Autodesk Fusion 360 part; units mm, degrees
(part 2 of 2)
extrude "Extrusion16" cut sketch "Esquisse2" along normal blind 100 contours L1 L2 L3 L4 A0 A1 A2 A3 | L9 L10 L11 L12 bodies 1 2
extrude "Extrusion17" add sketch "Esquisse3" against normal blind 1.4 contours L0 L1 L2 L3 | A0 L4 A1 L5 A2 L6 A3 L7 L288 L289 L290 L291 | A2 A6 | L8 L9 L10 L11 | L12 L13 L14 L15 | L16 L17 L18 L19 | L20 L21 L22 L23 | L24 L25 L26 L27 | L28 L29 L30 L31 | L32 L33 L34 L35 | L36 L37 L38 L39 | L40 L41 L42 L43 | L44 L45 L46 L47 | L48 L49 L50 L51 | L52 L53 L54 L55 | L56 L57 L58 L59 | L60 L61 L62 L63 | L64 L65 L66 L67 | L68 L69 L70 L71 | L72 L73 L74 L75 | L76 L77 L78 L79 | L80 L81 L82 L83 | L84 L85 L86 L87 | L88 L89 L90 L91 | L92 L93 L94 L95 | L96 L97 L98 L99 | L100 L101 L102 L103 | L104 L105 L106 L107 | L108 L109 L110 L111 | L112 L113 L114 L115 | L116 L117 L118 L119 | L120 L121 L122 L123 | L124 L125 L126 L127 | L128 L129 L130 L131 | L132 L133 L134 L135 | L136 L137 L138 L139 | L140 L141 L142 L143 | L144 L145 L146 L147 | L148 L149 L150 L151 | L152 L153 L154 L155 | L156 L157 L158 L159 | L160 L161 L162 L163 | L164 L165 L166 L167 | L168 L169 L170 L171 | L172 L173 L174 L175 | L176 L177 L178 L179 | L180 L182 L183 A9 | L180 A9 | L180 L182 A9 | L180 L181 L182 A9 | L182 A9 | L184 L185 L186 L187 | L188 L189 L190 L191 | L192 L193 L194 L195 | L196 L197 L198 L199 | L200 L201 L202 L203 | L204 L205 L206 L207 L208 L209 L210 L211 | L212 L213 L214 L215 | L216 L218 L219 A8 | L216 A8 | L216 L218 A8 | L216 L217 L218 A8 | L218 A8 | L220 L221 L222 L223 | L224 L225 L226 L227 | L228 L229 L230 L231 | L232 L233 L234 L235 | L236 L237 L238 L239 | L240 L241 L242 L243 | L244 L245 L246 L247 | L248 L249 L250 L251 | L252 L253 L254 L255 | L256 L257 L258 L259 | L260 L261 L262 L263 | L264 L265 L266 L267 | L268 L269 L270 L271 | L272 L273 L274 L275 | L276 L277 L278 L279 | L280 L281 L282 L283 | L284 L285 L286 L287 | A10 | A11 bodies 2
sketch "Esquisse4" plane through (0, 0, -17.4) normal (0, 0, -1) x (1, 0, 0)
  line L0 (-34.05, -60.68) -> (34.05, -60.68)
  arc A0 (34.05, -60.68) -> (36.05, -58.68) centre (33.45, -58.08) ccw
  line L1 (36.05, -58.68) -> (36.05, 58.68)
  arc A1 (36.05, 58.68) -> (34.05, 60.68) centre (34.05, 58.68) ccw
  line L2 (34.05, 60.68) -> (-34.05, 60.68)
  arc A2 (-34.05, 60.68) -> (-36.05, 58.68) centre (-33.45, 58.08) ccw
  line L3 (-36.05, 58.68) -> (-36.05, -58.68)
  arc A3 (-36.05, -58.68) -> (-34.05, -60.68) centre (-33.45, -58.08) ccw
  line L4 (-26.9549, 52.5905) -> (26.9549, 52.5905)
  line L5 (26.9549, 52.5905) -> (26.9549, -52.5905)
  line L6 (26.9549, -52.5905) -> (-26.9549, -52.5905)
  line L7 (-26.9549, -52.5905) -> (-26.9549, 52.5905)
  line L8 (-26.9549, 52.5905) -> (26.9549, -52.5905) construction
  line L9 (26.9549, 52.5905) -> (-26.9549, -52.5905) construction
  constraint horizontal L4
  constraint perpendicular L4 L5
  constraint parallel L4 L6
  constraint parallel L5 L7
  constraint coincident L8 origin
  constraint coincident L9 origin
extrude "Extrusion19" cut sketch "Esquisse2" along normal blind 74 contours L17 L18 L19 L20 bodies 2
extrude "Extrusion20" cut sketch "Esquisse1" against normal up to surface (6 mm away) from surface at -4 contours L321 L355 L361 L367 bodies 2
extrude "Extrusion21" add 1 faces at (35.4931, 59.8808, -16) along direction (0, 0, -1) up to surface (1.4 mm away) on bodies 2 bodies 2
extrude "Extrusion22" add 1 faces at (-35.4931, 59.8808, -16) along direction (0, 0, -1) up to surface (1.4 mm away) on bodies 2 bodies 2
extrude "Extrusion23" add 1 faces at (-35.2508, -60.1231, -16) along direction (0, 0, -1) up to surface (1.4 mm away) on bodies 2 bodies 2
extrude "Extrusion24" add sketch "Esquisse3" along normal blind 13.6 contours L180 A9 | L180 L182 A9 | L182 A9 | L216 A8 | L216 L218 A8 | L218 A8 bodies 2
extrude "Extrusion25" add sketch "Esquisse3" along normal blind 13.6 contours A10 | A11 bodies 2
sketch "Esquisse5" plane through (0, 0, 0) normal (0, 1, 0) x (1, 0, 0)
  line L0 (2.5, 5.4) -> (-2.5, 5.4)
  line L1 (-2.5, 5.4) -> (-2.5, 2.6)
  line L2 (-2.5, 2.6) -> (2.5, 2.6)
  line L3 (2.5, 2.6) -> (2.5, 5.4)
  line L4 (2.5, 5.4) -> (-2.5, 2.6) construction
  line L5 (-2.5, 5.4) -> (2.5, 2.6) construction
  point P0 (0, 4)
  point P1 (0, 4)
  dimension "d152" = 5
  dimension "d153" = 2.8
  constraint horizontal L0
  constraint perpendicular L0 L1
  constraint parallel L0 L2
  constraint parallel L1 L3
  constraint coincident L4 P1
  constraint coincident L5 P1
  constraint coincident P0 P1
  measures "d152" distance of L1.end L2.end
  measures "d153" distance of L0.end L1.end
extrude "Extrusion26" cut sketch "Esquisse5" along normal blind 1 from surface at -60.68 bodies 2
extrude "Extrusion27" cut sketch "Esquisse5" against normal blind 1 from surface at 60.68 bodies 2
extrude "Extrusion13" [suppressed]
equation "LongueurEPI = 115.36 mm"
equation "LargeurEPI = 66.10 mm"
equation "epaisseur = 2 mm"
equation "distance_bouton_largeur = 2.15 mm"
equation "erreur1 = 0.2 mm"
equation "hauteur_bouton = 5.6 mm"
equation "largeur_bouton = 4.5 mm"
equation "erreur_bouton = 0.2 mm"
equation "distance_bouton_hauteur = 1.91 mm"
equation "largeur_ecran = 63.5 mm"
equation "hauteur_ecran = 44.3 mm"
equation "d12 = LargeurEPI"
equation "d13 = LongueurEPI"
equation "d14 = largeur_ecran + erreur1"
equation "d15 = hauteur_ecran"
equation "d16 = distance_bord_ecran"
equation "distance_bord_ecran = 1.3 mm"
equation "bord_bas_touche = 3.3 mm"
equation "bord_cote_touche = 1.7 mm"
equation "d20 = 3.4 mm + hauteur_bouton / 2"
equation "d21 = distance_bouton_largeur / 2 + largeur_bouton / 2"
equation "d22 = largeur_bouton"
equation "d23 = hauteur_bouton"
equation "d26 = distance_bouton_largeur + largeur_bouton"
equation "d27 = hauteur_bouton + distance_bouton_hauteur"
equation "d36 = largeur_bouton"
equation "d37 = hauteur_bouton"
equation "d38 = largeur_bouton"
equation "d39 = hauteur_bouton"
equation "d42 = largeur_bouton"
equation "d43 = hauteur_bouton"
equation "d44 = largeur_bouton"
equation "d45 = hauteur_bouton"
equation "d48 = largeur_bouton"
equation "d49 = hauteur_bouton"
equation "profondeur_face = 1.4 mm"
equation "arrondi = 2 mm"
equation "largeur_USBC = 3.6 mm"
equation "longueur_USBC = 9.3 mm"
equation "d63 = longueur_USBC"
equation "d64 = largeur_USBC"
equation "largeur_ONOFF = 3.5 mm"
equation "longueur_ONOFF = 6.7 mm"
equation "d70 = longueur_ONOFF"
equation "d71 = largeur_ONOFF"
equation "marge_bord_epi = 0.4 mm"
equation "d81 = -marge_bord_epi"
equation "d83 = arrondi"
equation "d84 = profondeur_face"
equation "d88 = profondeur_face - 0.4 mm"
equation "cote_emboitement = 0.2 mm"
equation "epaisseur_boitier_epi = 16 mm"
equation "d94 = -epaisseur_boitier_epi"
equation "longueur_encoche_maintient = 10 mm"
equation "largeur_encoche_maintient = 1 mm"
equation "hauteur_encoche_maintient = 5.8 mm"
equation "d112 = -cote_emboitement"
equation "d113 = -cote_emboitement"
equation "d115 = -hauteur_encoche_maintient"
equation "d122 = -hauteur_encoche_maintient - 0.2 mm"
equation "d126 = -profondeur_face"
equation "d147 = 15 mm - profondeur_face"
equation "d150 = 15 mm - profondeur_face"
